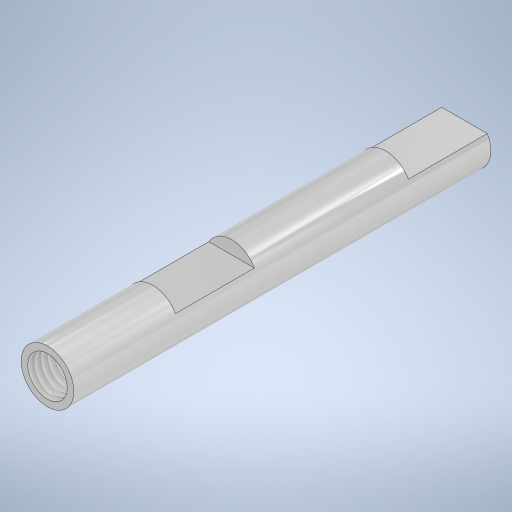
# Autodesk Inventor part: shaft_31.7mm_Dcut
Saved by Autodesk Inventor 2024 (Build 280153000, 153)
## iProperties
Created: 2025-05-27
Part Number: shaft_31.7mm_Dcut
Material: アルミニウム
Document SubType Name: Modeling
Designer: 1412z
Density: 2.7 g/cm^3
Appearance: アルミニウム - つや出し
Author: 1412z
Autodesk Inventor part; units mm, degrees
ref_plane "YZ Plane" through (0, 0, 0) normal (1, 0, 0) x (0, 1, 0)
ref_plane "XZ Plane" through (0, 0, 0) normal (0, 1, 0) x (-1, 0, 0)
ref_plane "XY Plane" through (0, 0, 0) normal (0, 0, 1) x (1, 0, 0)
sketch "スケッチ1" plane through (0, 0, 0) normal (1, 0, 0) x (0, 1, 0)
  line L0 (0, 0) -> (2, 0)
  line L1 (2, 0) -> (2, 31.7)
  line L2 (2, 31.7) -> (1.5, 31.7)
  line L3 (1.5, 31.7) -> (1.5, 25.7)
  line L4 (1.5, 25.7) -> (0, 25.7)
  line L5 (0, 25.7) -> (0, 0)
  dimension "d0" = 2
  dimension "d1" = 31.7
  dimension "d2" = 0.5
  dimension "d3" = 6
  constraints: 12 end point, 3 perpendicular, 2 horizontal, 1 parallel
  measures "d0" distance of L0.start L0.end
  measures "d1" distance of L0.end L1.end
  measures "d2" distance of L1.end L2.end
  measures "d3" distance of L2.end L3.end
revolve "回転1" add sketch "スケッチ1" angle 360 about axis through (0, 0, 25.7) along (0, 0, -1)
thread "ねじ1" size "M3x0.5" class "6H" standard "ANSI Metric M Profile" full length
sketch "スケッチ2" plane through (0, 0, 0) normal (1, 0, 0) x (0, 1, 0)
  line L0 (2, 31.7) -> (2, 0) projected
  line L1 (2, 0) -> (2, 6)
  line L2 (2, 6) -> (1, 6)
  line L3 (1, 6) -> (1, 0)
  line L4 (-2, 0) -> (2, 0) projected
  line L5 (1, 0) -> (2, 0)
  point P0 (0, 0)
  dimension "d7" = 6
  dimension "d8" = 1
  constraints: 8 end point, 3 point on line, 2 perpendicular, 1 horizontal
  measures "d7" distance of L1.start L1.end
  measures "d8" distance of L1.end L2.end
extrude "押し出し1" cut sketch "スケッチ2" along normal mid plane 6
sketch "スケッチ3" plane through (0, 0, 0) normal (1, 0, 0) x (0, 1, 0)
  line L0 (2, 31.7) -> (2, 6) projected
  line L1 (2, 20.7) -> (2, 23.7)
  line L2 (2, 23.7) -> (1, 23.7)
  line L3 (1, 23.7) -> (1, 17.7)
  line L4 (1, 17.7) -> (2, 17.7)
  line L5 (2, 17.7) -> (2, 20.7)
  point P0 (0, 0)
  dimension "d11" = 3
  dimension "d12" = 1
  dimension "d13" = 6
  constraints: 10 end point, 4 perpendicular, 3 point on line
  measures "d11" distance of L1.start L1.end
  measures "d12" distance of L1.end L2.end
  measures "d13" distance of L2.end L3.end
extrude "押し出し2" cut sketch "スケッチ3" along normal mid plane 6
